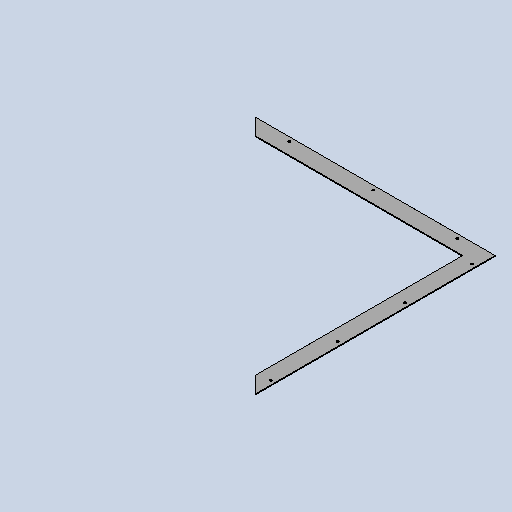
# Autodesk Inventor part: PNS waste water bin 01
Saved by Autodesk Inventor 2025.3 (Build 293356030, 356C)
## iProperties
Created: 2025-09-03
Part Number: PNS waste water bin 01
Material: Generic
Document SubType Name: Sheet Metal
Designer: admin
Density: 1 g/cm^3
Appearance: Default
Sheet Metal Rule: Default
Flat Pattern Width: 56.9293 cm
Flat Pattern Length: 56.9293 cm
Flat Pattern Area: 3240.94 cm^2
Sheet Metal Width: 569,293 mm
Sheet Metal Length: 569,293 mm
Sheet Metal Area: 324094,398 mm^2
Mass: 81.517 g
Surface Area: 862.237 cm^2
Volume: 81.517 cm^3
Author: admin
Autodesk Inventor part; units mm, degrees
ref_plane "YZ Plane" through (0, 0, 0) normal (1, 0, 0) x (0, 1, 0)
ref_plane "XZ Plane" through (0, 0, 0) normal (0, 1, 0) x (-1, 0, 0)
ref_plane "XY Plane" through (0, 0, 0) normal (0, 0, 1) x (1, 0, 0)
sketch "Sketch1" plane through (0, 0, 0) normal (0, 0, 1) x (1, 0, 0)
  line L0 (-285, 285) -> (285, 285)
  line L1 (285, 285) -> (285, -285)
  line L2 (285, -285) -> (-285, -285)
  line L3 (-285, -285) -> (-285, 285)
  line L4 (-285, 285) -> (285, -285) construction
  line L5 (285, 285) -> (-285, -285) construction
  line L6 (-246.5, -246.5) -> (246.5, -246.5)
  line L7 (246.5, -246.5) -> (246.5, 246.5)
  line L8 (246.5, 246.5) -> (-246.5, 246.5)
  line L9 (-246.5, 246.5) -> (-246.5, -246.5)
  line L10 (-246.5, -246.5) -> (246.5, 246.5) construction
  line L11 (246.5, -246.5) -> (-246.5, 246.5) construction
  line L12 (-246.5, 246.5) -> (-285, 285)
  line L13 (246.5, -246.5) -> (285, -285)
  point P0 (0, 0)
  dimension "d1" = 570
  dimension "d2" = 493
  measures "d1" distance of L0.end L1.end
  measures "d2" distance of L8.end L7.end
extrude "Plate1" add sketch "Sketch1" along normal blind 2 contours L0 L1 L13 L7 L8 L12
chamfer "Corner Chamfer1" distance 1 angle 45 2 edges at (-285, 285, 1) (285, -285, 1)
sketch "Sketch2" plane through (0, 0, 0) normal (0, 0, -1) x (-1, 0, 0)
  line L0 (-284.2929, -284.2929) -> (-285, -284) projected
  line L1 (-246.5, -246.5) -> (-284.2929, -284.2929) projected
  line L2 (-246.5, 246.5) -> (-246.5, -246.5) construction
  line L3 (246.5, 246.5) -> (-246.5, 246.5) construction
  line L4 (284.2929, 284.2929) -> (246.5, 246.5) projected
  line L5 (284, 285) -> (284.2929, 284.2929) projected
  line L6 (-285, 285) -> (284, 285) construction
  line L7 (-285, -284) -> (-285, 285) construction
  circle A0 centre (-275, 240.5) radius 2.75
  circle A1 centre (-275, 80.5) radius 2.75
  circle A2 centre (-275, -79.5) radius 2.75
  circle A3 centre (-275, -239.5) radius 2.75
  line L8 (-275, 285) -> (-275, -275) construction
  line L9 (-285, 275) -> (275, 275) construction
  line L10 (-285, -284) -> (-285, 285) construction
  circle A4 centre (-205, 275) radius 2.75
  circle A5 centre (-5, 275) radius 2.75
  circle A6 centre (195, 275) radius 2.75
  point P0 (0, 0)
  point P1 (-285, 0.5)
  point P2 (-285, 0.5)
  point P3 (-285, 0.5)
  point P4 (-285, 0.5)
  dimension "d7" = 5.5
  dimension "d8" = 10
  dimension "d9" = 10
  dimension "d10" = 80
  dimension "d11" = 80
  dimension "d12" = 240
  dimension "d13" = 240
  dimension "d14" = 200
  dimension "d15" = 200
  constraints: 10 point on line, 7 centre point, 6 equal radius, 5 midpoint, 4 end point, 2 parallel
  measures "d7" diameter of A0
  measures "d8" distance between parallel lines of L6 L9
  measures "d9" distance between parallel lines of L7 L8
  measures "d10" vertical distance of A1.centre point (-285, 0.5)
  measures "d11" vertical distance of A2.centre point (-285, 0.5)
  measures "d12" vertical distance of A0.centre point (-285, 0.5)
  measures "d13" vertical distance of A3.centre point (-285, 0.5)
  measures "d14" distance of A5.centre A4.centre
  measures "d15" distance of A5.centre A6.centre
extrude "Cut1" cut sketch "Sketch2" against normal blind 2
equation "\"d9\" = d8"
equation "\"d11\" = d10"
equation "\"d13\" = d12"
equation "\"d15\" = d14"
equation "\"d16\" = Thickness"
equation "\"d3\" = Thickness"
equation "\"BendRadius\" = Thickness"
equation "\"BendReliefWidth\" = Thickness"
equation "\"BendReliefDepth\" = 0.5 * Thickness"
equation "\"CornerReliefSize\" = 4 * Thickness"
equation "\"MinimumRemnant\" = 2 * Thickness"
equation "\"TransitionRadius\" = BendRadius"
equation "\"JacobiRadiusSize\" = BendRadius"
equation "\"GapSize\" = Thickness"
equation "\"Thickness\" = 2"
body "Solid1"
